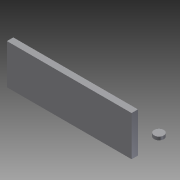
# Autodesk Inventor part: DB15 connector
Saved by Autodesk Inventor 2012 (Build 160160000, 160)
## iProperties
Created: 2017-04-26
Part Number: DB15 connector
Material: Default
Document SubType Name: Modeling
Designer: Brandon
Density: 1 g/cm^3
Author: Brandon
Autodesk Inventor part; units mm, degrees
ref_plane "YZ Plane" through (0, 0, 0) normal (1, 0, 0) x (0, 1, 0)
ref_plane "XZ Plane" through (0, 0, 0) normal (0, 1, 0) x (-1, 0, 0)
ref_plane "XY Plane" through (0, 0, 0) normal (0, 0, 1) x (1, 0, 0)
sketch "Sketch1" plane through (0, 0, 0) normal (0, 0, 1) x (1, 0, 0)
  line L0 (-19.57, 12.55) -> (19.57, 12.55)
  line L1 (19.57, 12.55) -> (19.57, 0)
  line L2 (19.57, 0) -> (-19.57, 0)
  line L3 (-19.57, 0) -> (-19.57, 12.55)
  point P0 (0, 0)
  dimension "d0" = 39.14
  dimension "d1" = 12.55
  dimension "d2" = 19.57
  dimension "d3" = 0
  constraints: 8 end point, 2 parallel, 1 horizontal, 1 perpendicular
  measures "d0" distance of L1.end L2.end
  measures "d1" distance of L0.end L1.end
  measures "d2" distance from line of point (0, 0) L1
  measures "d3" distance from line of L2 point (0, 0)
extrude "Extrusion1" add sketch "Sketch1" along normal blind 2
sketch "Sketch2" plane through (-19.57, 0, 0) normal (0, -1, 0) x (1, 0, 0)
  line L0 (39.14, 0) -> (0, 0) projected
  circle A0 centre (2.91, -9.5) radius 1.525
  circle A1 centre (36.23, -9.5) radius 1.525
  point P0 (19.57, 0)
  dimension "d6" = 3.05
  dimension "d7" = 3.05
  dimension "d8" = 33.32
  dimension "d9" = 16.66
  dimension "d10" = 9.5
  dimension "d11" = 9.5
  constraints: 2 centre point
  measures "d6" diameter of A0
  measures "d7" diameter of A1
  measures "d8" distance of A1.centre A0.centre
  measures "d9" horizontal distance of point (19.57, 0) A1.centre
  measures "d10" distance from line of L0 A0.centre
  measures "d11" distance from line of L0 A1.centre
extrude "Extrusion2" add sketch "Sketch2" along normal blind 1
equation "\"d2\" = 0.5 * d0"
equation "\"d9\" = 0.5 * d8"
body "Solid1"
